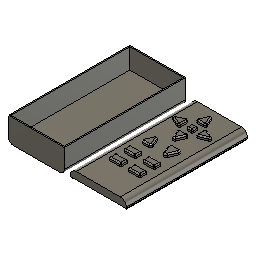
northreach_1_v1 (Autodesk Fusion 360 design; units mm, degrees)
Autodesk Fusion 360 part; units mm, degrees
sketch "Sketch1" plane through (0, 0, 0) normal (0, 1, 0) x (1, 0, 0)
  line L0 (-22.5, 50) -> (22.5, 50)
  line L1 (22.5, 50) -> (22.5, -50)
  line L2 (22.5, -50) -> (-22.5, -50)
  line L3 (-22.5, -50) -> (-22.5, 50)
  line L4 (-22.5, 50) -> (22.5, -50) construction
  line L5 (22.5, 50) -> (-22.5, -50) construction
  line L6 (-23.5, 51) -> (23.5, 51)
  line L7 (23.5, 51) -> (23.5, -51)
  line L8 (23.5, -51) -> (-23.5, -51)
  line L9 (-23.5, -51) -> (-23.5, 51)
  line L10 (-23.5, 51) -> (23.5, -51) construction
  line L11 (23.5, 51) -> (-23.5, -51) construction
  dimension "d1" = 45
  dimension "d2" = 100
  dimension "d3" = 47
  dimension "d4" = 102
  constraint horizontal L0
  constraint perpendicular L0 L1
  constraint parallel L0 L2
  constraint parallel L1 L3
  constraint coincident L4 origin
  constraint coincident L5 origin
  constraint horizontal L6
  constraint perpendicular L6 L7
  constraint parallel L6 L8
  constraint parallel L7 L9
  constraint coincident L10 origin
  constraint coincident L11 origin
  measures "d1" distance of L1.end L2.end
  measures "d2" distance of L0.end L1.end
  measures "d3" distance of L7.end L8.end
  measures "d4" distance of L6.end L7.end
extrude "Extrude1" add sketch "Sketch1" along normal blind 3 contours L0 L1 L2 L3 makes body 1
extrude "Extrude2" add sketch "Sketch1" along normal blind 20 bodies 1
fillet "Fillet1" radius 4 2 edges at (-23.5, 0, 0) (23.5, 0, 0) on bodies 1
sketch "Sketch4" plane through (0, 0, 0) normal (0, 1, 0) x (1, 0, 0)
  line L0 (46.5, 51) -> (93.5, 51)
  line L1 (93.5, 51) -> (93.5, -51)
  line L2 (93.5, -51) -> (46.5, -51)
  line L3 (46.5, -51) -> (46.5, 51)
  line L4 (46.5, 51) -> (93.5, -51) construction
  line L5 (93.5, 51) -> (46.5, -51) construction
  line L6 (48.5, 50) -> (91.5, 50)
  line L7 (91.5, 50) -> (91.5, -50)
  line L8 (91.5, -50) -> (48.5, -50)
  line L9 (48.5, -50) -> (48.5, 50)
  line L10 (48.5, 50) -> (91.5, -50) construction
  line L11 (91.5, 50) -> (48.5, -50) construction
  line L12 (48.5, 50) -> (47.5, 50)
  line L13 (47.5, 50) -> (47.5, -50)
  line L14 (47.5, -50) -> (48.5, -50)
  line L15 (48.5, -50) -> (48.5, 50)
  line L16 (91.5, -50) -> (92.5, -50)
  line L17 (92.5, -50) -> (92.5, 50)
  line L18 (92.5, 50) -> (91.5, 50)
  line L19 (91.5, 50) -> (91.5, -50)
  point P0 (70, 0)
  point P1 (70, 0)
  dimension "d22" = 47
  dimension "d23" = 102
  dimension "d24" = 43
  dimension "d25" = 100
  constraint horizontal L0
  constraint perpendicular L0 L1
  constraint parallel L0 L2
  constraint parallel L1 L3
  constraint coincident L4 P1
  constraint coincident L5 P1
  constraint horizontal L6
  constraint perpendicular L6 L7
  constraint parallel L6 L8
  constraint parallel L7 L9
  constraint coincident L10 P1
  constraint coincident L11 P1
  constraint coincident P1 P0
  constraint horizontal L12
  constraint vertical L13
  constraint horizontal L14
  constraint vertical L15
  constraint horizontal L16
  constraint vertical L17
  constraint horizontal L18
  constraint vertical L19
  measures "d22" distance of L1.end L2.end
  measures "d23" distance of L0.end L1.end
  measures "d24" distance of L7.end L8.end
  measures "d25" distance of L6.end L7.end
extrude "Extrude7" add sketch "Sketch4" along normal blind 2 separate body contours L6 L7 L8 L9 L15 L19 makes body 2
extrude "Extrude8" add sketch "Sketch4" along normal blind 6 bodies 2
extrude "Extrude9" add sketch "Sketch4" along normal blind 7.5 contours L9 L12 L13 L14 L15 | L7 L16 L17 L18 L19 bodies 2
fillet "Fillet2" radius 5 4 edges at (91.5, 2, 0) (48.5, 2, 0) (46.5, 0, 0) (93.5, 0, 0) on bodies 2
move_body "Move1" bodies 2 to x (-1, 0, 0) y (0, -1, 0) z (0, 0, 1) at (122, 7.5, 0)
sketch "Sketch5" plane through (0, 7.5, 0) normal (0, 1, 0) x (-1, 0, 0)
  line L0 (-33.5, -51) -> (-33.5, 51)
  line L1 (-33.5, 51) -> (-70.5, 51)
  line L2 (-70.5, 51) -> (-70.5, -51)
  line L3 (-70.5, -51) -> (-33.5, -51)
  arc A0 (-59.0385, -25.2061) -> (-60.6066, -24.1721) centre (-60.1635, -25.2061) ccw
  arc A1 (-39, 16.25) -> (-39.75, 17) centre (-39.75, 16.25) ccw
  line L4 (-49, 14) -> (-55, 14)
  arc A2 (-50.25, -30.5) -> (-49.5, -29.75) centre (-50.25, -29.75) ccw
  line L5 (-39.75, 11) -> (-48.25, 11)
  arc A3 (-55, 16.25) -> (-55.75, 17) centre (-55.75, 16.25) ccw
  line L6 (-46, 14) -> (-42, 14)
  line L7 (-53.75, -30.5) -> (-50.25, -30.5)
  arc A4 (-36.8743, -29.034) -> (-36.8743, -26.966) centre (-37.3174, -28) ccw
  line L8 (-54.5, -26.25) -> (-54.5, -29.75)
  line L9 (-49.5, -25.5) -> (-54.5, -30.5) construction
  arc A5 (-65, 11.75) -> (-64.25, 11) centre (-64.25, 11.75) ccw
  arc A6 (-49.2061, -20.9615) -> (-48.1721, -19.3934) centre (-49.2061, -19.8365) ccw
  line L10 (-65, 11) -> (-55, 17) construction
  line L11 (-39, 16.25) -> (-39, 11.75)
  line L12 (-48.25, 17) -> (-39.75, 17)
  line L13 (-65, 23) -> (-55, 29) construction
  line L14 (-62, 26) -> (-58, 26)
  line L15 (-41.4931, 3.0384) -> (-46.5069, 3.0384)
  line L16 (-39, 28.25) -> (-39, 23.75)
  arc A7 (-57.46, -6.6101) -> (-55.6908, -3.9272) centre (-57.46, -4.6854) ccw
  line L17 (-55.75, 23) -> (-64.25, 23)
  arc A8 (-39.75, 11) -> (-39, 11.75) centre (-39.75, 11.75) ccw
  line L18 (-49, 23) -> (-39, 29) construction
  line L19 (-39.75, 23) -> (-48.25, 23)
  arc A9 (-64.25, 29) -> (-65, 28.25) centre (-64.25, 28.25) ccw
  line L20 (-60, -6.6101) -> (-60, 3.4562)
  arc A10 (-64.3092, -3.9272) -> (-62.54, -6.6101) centre (-62.54, -4.6854) ccw
  arc A11 (-48.1721, -36.6066) -> (-49.2061, -35.0385) centre (-49.2061, -36.1635) ccw
  line L21 (-55, 11) -> (-65, 17) construction
  arc A12 (-49.5, -26.25) -> (-50.25, -25.5) centre (-50.25, -26.25) ccw
  line L22 (-49, 11) -> (-39, 17) construction
  arc A13 (-54.7939, -35.0385) -> (-55.8279, -36.6066) centre (-54.7939, -36.1635) ccw
  arc A14 (-49, 23.75) -> (-48.25, 23) centre (-48.25, 23.75) ccw
  line L23 (-47.8763, 0.9617) -> (-45.1295, -5.4475)
  arc A15 (-50.966, -12.8743) -> (-53.034, -12.8743) centre (-52, -13.3174) ccw
  line L24 (-58.4041, 2.4038) -> (-55.6908, -3.9272)
  arc A16 (-55.8279, -19.3934) -> (-54.7939, -20.9615) centre (-54.7939, -19.8365) ccw
  line L25 (-55, 28.25) -> (-55, 23.75)
  line L26 (-36.8743, -29.034) -> (-43.3934, -31.8279)
  arc A17 (-67.1257, -26.966) -> (-67.1257, -29.034) centre (-66.6826, -28) ccw
  line L27 (-49, 26) -> (-55, 26)
  line L28 (-57.46, -6.6101) -> (-62.54, -6.6101)
  line L29 (-50.966, -12.8743) -> (-48.1721, -19.3934)
  arc A18 (-47.8763, 0.9617) -> (-46.5069, 3.0384) centre (-46.5069, 1.5486) cw
  arc A19 (-58.4041, 2.4038) -> (-61.5959, 2.4038) centre (-60, 1.7199) ccw
  line L30 (-42.8705, -5.4475) -> (-40.1237, 0.9617)
  arc A20 (-36.8743, -29.034) -> (-36.8743, -26.966) centre (-37.3174, -28) ccw
  line L31 (-55, 23) -> (-65, 29) construction
  arc A21 (-55, 28.25) -> (-55.75, 29) centre (-55.75, 28.25) ccw
  line L32 (-54.5, -25.5) -> (-49.5, -30.5) construction
  line L33 (-36.8743, -29.034) -> (-43.3934, -31.8279)
  line L34 (-44.9615, -30.7939) -> (-44.9615, -25.2061)
  arc A22 (-44.9615, -30.7939) -> (-43.3934, -31.8279) centre (-43.8365, -30.7939) ccw
  line L35 (-65, 23.75) -> (-65, 28.25)
  line L36 (-46, 26) -> (-42, 26)
  line L37 (-64.25, 17) -> (-55.75, 17)
  line L38 (-59.0385, -25.2061) -> (-59.0385, -30.7939)
  line L39 (-39, 11) -> (-49, 17) construction
  arc A23 (-54.5, -29.75) -> (-53.75, -30.5) centre (-53.75, -29.75) ccw
  line L40 (-67.1257, -26.966) -> (-60.6066, -24.1721)
  line L41 (-43.3934, -24.1721) -> (-36.8743, -26.966)
  line L42 (-60.6066, -31.8279) -> (-67.1257, -29.034)
  line L43 (-50.25, -25.5) -> (-53.75, -25.5)
  arc A24 (-53.75, -25.5) -> (-54.5, -26.25) centre (-53.75, -26.25) ccw
  line L44 (-48.1721, -36.6066) -> (-50.966, -43.1257)
  line L45 (-49.2061, -20.9615) -> (-54.7939, -20.9615)
  line L46 (-44, 12) -> (-44, 16)
  arc A25 (-49, 11.75) -> (-48.25, 11) centre (-48.25, 11.75) ccw
  line L47 (-60, 24) -> (-60, 28)
  line L48 (-65, 11.75) -> (-65, 16.25)
  line L49 (-44, 24) -> (-44, 28)
  line L50 (-39, 23) -> (-49, 29) construction
  arc A26 (-43.3934, -24.1721) -> (-44.9615, -25.2061) centre (-43.8365, -25.2061) ccw
  line L51 (-62, 14) -> (-58, 14)
  line L52 (-49.5, -29.75) -> (-49.5, -26.25)
  line L53 (-60, 12) -> (-60, 16)
  arc A27 (-64.25, 17) -> (-65, 16.25) centre (-64.25, 16.25) ccw
  line L54 (-49, 11.75) -> (-49, 16.25)
  arc A28 (-65, 23.75) -> (-64.25, 23) centre (-64.25, 23.75) ccw
  arc A29 (-53.034, -43.1257) -> (-50.966, -43.1257) centre (-52, -42.6826) ccw
  arc A30 (-41.4931, 3.0384) -> (-40.1237, 0.9617) centre (-41.4931, 1.5486) cw
  arc A31 (-43.3934, -24.1721) -> (-44.9615, -25.2061) centre (-43.8365, -25.2061) ccw
  arc A32 (-48.25, 17) -> (-49, 16.25) centre (-48.25, 16.25) ccw
  arc A33 (-39, 28.25) -> (-39.75, 29) centre (-39.75, 28.25) ccw
  arc A34 (-44.9615, -30.7939) -> (-43.3934, -31.8279) centre (-43.8365, -30.7939) ccw
  line L55 (-44, -6.1923) -> (-44, 3.0384)
  line L56 (-49, 23.75) -> (-49, 28.25)
  line L57 (-43.3934, -24.1721) -> (-36.8743, -26.966)
  arc A35 (-55.75, 11) -> (-55, 11.75) centre (-55.75, 11.75) ccw
  arc A36 (-39.75, 23) -> (-39, 23.75) centre (-39.75, 23.75) ccw
  arc A37 (-60.6066, -31.8279) -> (-59.0385, -30.7939) centre (-60.1635, -30.7939) ccw
  line L58 (-48.25, 29) -> (-39.75, 29)
  line L59 (-54.7939, -35.0385) -> (-49.2061, -35.0385)
  line L60 (-55.75, 11) -> (-64.25, 11)
  line L61 (-44.9615, -30.7939) -> (-44.9615, -25.2061)
  line L62 (-55.8279, -19.3934) -> (-53.034, -12.8743)
  arc A38 (-48.25, 29) -> (-49, 28.25) centre (-48.25, 28.25) ccw
  line L63 (-53.034, -43.1257) -> (-55.8279, -36.6066)
  arc A39 (-42.8705, -5.4475) -> (-45.1295, -5.4475) centre (-44, -4.9635) cw
  line L64 (-64.3092, -3.9272) -> (-61.5959, 2.4038)
  line L65 (-64.25, 29) -> (-55.75, 29)
  arc A40 (-55.75, 23) -> (-55, 23.75) centre (-55.75, 23.75) ccw
  line L66 (-55, 16.25) -> (-55, 11.75)
  line L67 (-42, 16) -> (-46, 16) construction
  line L68 (-46, 16) -> (-46, 12) construction
  line L69 (-46, 12) -> (-42, 12) construction
  line L70 (-42, 12) -> (-42, 16) construction
  line L71 (-42, 28) -> (-46, 28) construction
  line L72 (-46, 28) -> (-46, 24) construction
  line L73 (-46, 24) -> (-42, 24) construction
  line L74 (-42, 24) -> (-42, 28) construction
  line L75 (-58, 16) -> (-62, 16) construction
  line L76 (-62, 16) -> (-62, 12) construction
  line L77 (-62, 12) -> (-58, 12) construction
  line L78 (-58, 12) -> (-58, 16) construction
  line L79 (-58, 28) -> (-62, 28) construction
  line L80 (-62, 28) -> (-62, 24) construction
  line L81 (-62, 24) -> (-58, 24) construction
  line L82 (-58, 24) -> (-58, 28) construction
  line L83 (-52, -35.0385) -> (-52, -43.8076)
  line L84 (-59.0385, -28) -> (-67.8076, -28)
  line L85 (-36.1924, -28) -> (-44.9615, -28)
  line L86 (-52, -20.9615) -> (-52, -12.1924)
  line L87 (-44, -1.577) -> (-60, -1.577)
  point P0 (-44, 26)
  point P1 (-60, 14)
  point P2 (-44, 3.0384)
  point P3 (-52.0007, 8.4459)
  point P4 (-44, 14)
  point P5 (-60, -6.6101)
  point P6 (-41.5, 10)
  point P7 (-44, 14)
  point P8 (-41.5, 22)
  point P9 (-44, 26)
  point P10 (-52, 14)
  point P11 (-60, -1.577)
  point P12 (-44, -1.577)
  point P13 (-52, 26)
  point P14 (-60, 14)
  point P15 (-52, -28)
  point P16 (-60, 26)
  point P17 (-60, 26)
  point P18 (-52, -39.423)
  point P19 (-63.423, -28)
  point P20 (-52, -16.577)
  point P21 (-40.577, -28)
  point P22 (-52, -1.577)
  dimension "d46" = 3
  dimension "d47" = 0
  dimension "d50" = 3
  dimension "d51" = 0
  dimension "d48" = 3
  dimension "d49" = 0
  dimension "d52" = 3
  dimension "d53" = 0
  dimension "d55" = 0.75
  dimension "d56" = 10
  dimension "d57" = 6
  dimension "d58" = 10
  dimension "d59" = 6
  dimension "d60" = 6
  dimension "d61" = 0.75
  dimension "d62" = 10
  dimension "d63" = 6
  dimension "d64" = 10
  dimension "d65" = 6
  dimension "d66" = 6
  dimension "d67" = 0.75
  dimension "d73" = 16
  text T0 "1" font "Arial" height 3 align centre middle in box 4 x 4 at (-42, 16) x (-1, 0) y (0, -1) spacing 1 kerned
  text T1 "3" font "Arial" height 3 align centre middle in box 4 x 4 at (-42, 28) x (-1, 0) y (0, -1) spacing 1 kerned
  text T2 "2" font "Arial" height 3 align centre middle in box 4 x 4 at (-58, 16) x (-1, 0) y (0, -1) spacing 1 kerned
  text T3 "4" font "Arial" height 3 align centre middle in box 4 x 4 at (-58, 28) x (-1, 0) y (0, -1) spacing 1 kerned
  constraint vertical L61
  constraint tangent L44 A29
  constraint tangent A29 L63
  constraint tangent A13 L59
  constraint tangent A13 L63
  constraint equal A13 A29
  constraint tangent A11 L44
  constraint tangent A11 L59
  constraint equal A11 A29
  constraint tangent A34 L61
  constraint tangent L33 A34
  constraint tangent A26 L61
  constraint tangent A26 L57
  constraint tangent A4 L57
  constraint tangent A4 L33
  constraint tangent L38 A37
  constraint tangent L42 A37
  constraint tangent A0 L38
  constraint tangent A0 L40
  constraint tangent A17 L40
  constraint tangent A17 L42
  constraint tangent A16 L45
  constraint tangent A16 L62
  constraint tangent A6 L45
  constraint tangent A6 L29
  constraint tangent A15 L62
  constraint tangent A15 L29
  constraint vertical L34
  constraint tangent L34 A22
  constraint tangent L26 A22
  constraint tangent L34 A31
  constraint tangent L41 A31
  constraint tangent A20 L41
  constraint tangent L26 A20
  constraint horizontal L43
  constraint perpendicular L8 L43
  constraint parallel L7 L43
  constraint parallel L8 L52
  constraint coincident P15 L9
  constraint coincident P15 L32
  constraint coincident L9.end L7
  constraint coincident L9.end L8
  constraint tangent L7 A23
  constraint tangent L8 A23
  constraint coincident L32.end L7
  constraint coincident L32.end L52
  constraint tangent A2 L7
  constraint tangent A2 L52
  constraint equal A2 A23
  constraint coincident L9.start L52
  constraint coincident L9.start L43
  constraint tangent A12 L52
  constraint tangent A12 L43
  constraint equal A12 A23
  constraint coincident L32.start L43
  constraint coincident L32.start L8
  constraint tangent L43 A24
  constraint tangent L8 A24
  constraint equal A23 A24
  constraint tangent L15 A18
  constraint tangent L23 A18
  constraint tangent L15 A30
  constraint tangent L30 A30
  constraint tangent L23 A39
  constraint tangent L30 A39
  constraint midpoint P2 L15
  constraint tangent A10 L28
  constraint tangent A10 L64
  constraint tangent A7 L28
  constraint tangent A7 L24
  constraint tangent A19 L64
  constraint tangent L24 A19
  constraint midpoint P5 L28
  constraint midpoint L55.start A39
  constraint coincident P2 L55.end
  constraint perpendicular L15 L55
  constraint coincident P5 L20.start
  constraint midpoint L20.end A19
  constraint perpendicular L20 L28
  constraint midpoint P11 L20
  constraint midpoint P12 L55
  constraint horizontal L60
  constraint perpendicular L48 L60
  constraint parallel L37 L60
  constraint parallel L48 L66
  constraint horizontal L5
  constraint perpendicular L5 L54
  constraint parallel L5 L12
  constraint parallel L11 L54
  constraint midpoint P10 L4
  constraint tangent L11 A8
  constraint tangent L5 A8
  constraint tangent A1 L11
  constraint tangent A1 L12
  constraint equal A1 A8
  constraint coincident L4.start L54
  constraint tangent L12 A32
  constraint tangent L54 A32
  constraint equal A8 A32
  constraint tangent L5 A25
  constraint tangent A25 L54
  constraint equal A8 A25
  constraint coincident L4.end L66
  constraint coincident L21.start L66
  constraint tangent A35 L60
  constraint tangent A35 L66
  constraint equal A8 A35
  constraint coincident L10.end L66
  constraint tangent A3 L66
  constraint tangent A3 L37
  constraint equal A3 A8
  constraint coincident L21.end L37
  constraint tangent L37 A27
  constraint tangent L48 A27
  constraint equal A8 A27
  constraint tangent A5 L60
  constraint tangent A5 L48
  constraint equal A5 A8
  constraint horizontal L17
  constraint perpendicular L17 L35
  constraint parallel L17 L65
  constraint parallel L25 L35
  constraint horizontal L19
  constraint perpendicular L19 L56
  constraint parallel L19 L58
  constraint parallel L16 L56
  constraint midpoint P13 L27
  constraint tangent L16 A36
  constraint tangent L19 A36
  constraint tangent L16 A33
  constraint tangent A33 L58
  constraint equal A33 A36
  constraint coincident L27.start L56
  constraint tangent L58 A38
  constraint tangent L56 A38
  constraint equal A36 A38
  constraint tangent L19 A14
  constraint tangent A14 L56
  constraint equal A14 A36
  constraint coincident L27.end L25
  constraint coincident L31.start L25
  constraint tangent L17 A40
  constraint tangent L25 A40
  constraint equal A36 A40
  constraint coincident L13.end L25
  constraint tangent L25 A21
  constraint tangent A21 L65
  constraint equal A21 A36
  constraint coincident L31.end L65
  constraint tangent A9 L65
  constraint tangent A9 L35
  constraint equal A9 A36
  constraint tangent L17 A28
  constraint tangent L35 A28
  constraint equal A28 A36
  constraint midpoint L46.start L69
  constraint midpoint L46.end L67
  constraint midpoint L6.start L68
  constraint midpoint L6.end L70
  constraint midpoint P7 L6
  constraint midpoint L53.start L77
  constraint midpoint L53.end L75
  constraint midpoint L51.start L76
  constraint midpoint L51.end L78
  constraint midpoint P14 L51
  constraint midpoint L49.start L73
  constraint midpoint L49.end L71
  constraint midpoint L36.start L72
  constraint midpoint L36.end L74
  constraint midpoint P9 L36
  constraint midpoint L47.start L81
  constraint midpoint L47.end L79
  constraint midpoint L14.start L80
  constraint midpoint L14.end L82
  constraint midpoint P17 L14
  constraint midpoint L59 L83.start
  constraint midpoint A29 L83.end
  constraint perpendicular L59 L83
  constraint midpoint L83 P18
  constraint midpoint L38 L84.start
  constraint midpoint A17 L84.end
  constraint perpendicular L38 L84
  constraint midpoint L84 P19
  constraint midpoint A20 L85.start
  constraint midpoint L34 L85.end
  constraint perpendicular L34 L85
  constraint midpoint L45 L86.start
  constraint midpoint A15 L86.end
  constraint perpendicular L45 L86
  constraint midpoint L86 P20
  constraint midpoint L85 P21
  constraint coincident P12 L87.start
  constraint coincident P11 L87.end
  constraint perpendicular L20 L87
  constraint midpoint L87 P22
  measures "d55" radius of A23
  measures "d56" distance of L21.end L10.end
  measures "d57" distance of L21.end L10.start
  measures "d58" distance of L22.end L39.end
  measures "d59" distance of L22.start L39.end
  measures "d60" distance of L54 L66
  measures "d61" radius of A8
  measures "d62" distance of L13.end L31.end
  measures "d63" distance of L13.start L31.end
  measures "d64" distance of L50.end L18.end
  measures "d65" distance of L50.end L18.start
  measures "d66" distance of L25 L56
  measures "d67" radius of A36
  measures "d73" distance of P12 P11
extrude "Extrude10" add sketch "Sketch5" sketch "Sketch5" along normal blind 2.5 contours A0 A17 L38 L40 L84 | A17 L38 L42 A37 L84 | A1 L5 L11 L12 A8 A25 L54 A32 | A2 L7 L8 A12 A23 L43 A24 L52 | A3 A5 L37 L48 A27 A35 L60 L66 | A4 L26 A20 L33 L34 A22 A34 L61 L85 | A4 A20 L34 L41 A26 A31 L57 L61 L85 | A6 A15 L29 L45 L86 | A15 A16 L45 L62 L86 | L15 L30 A30 L55 A39 | L15 L23 A18 L55 L87 | L23 L55 A39 L87 | L16 L19 A14 A33 L56 A36 L58 A38 | A7 L20 L24 L28 L87 | L20 A10 L28 A19 L64 | L20 L24 A19 L87 | L17 A9 L25 A21 L35 A28 L65 A40 | A11 L44 A29 L59 L83 | A13 A29 L59 L63 L83 of sketch 2 text T0 T1 T2 T3 bodies 2
fillet "Fillet3" radius 1 76 edges at (52, 10, -35.0385) (55.7331, 10, -35.5442) (54.431, 10, -39.8662) (52, 10, -43.8076) (49.569, 10, -39.8662) (48.2669, 10, -35.5442) (40.1338, 10, -25.569) (44.4558, 10, -24.2669) (44.9615, 10, -28) (44.4558, 10, -31.7331) (40.1338, 10, -30.431) (36.1924, 10, -28) (63.8662, 10, -25.569) (67.8076, 10, -28) (63.8662, 10, -30.431) (59.5442, 10, -31.7331) (59.0385, 10, -28) (59.5442, 10, -24.2669) (54.2803, 10, -30.2803) (52, 10, -30.5) (49.7197, 10, -30.2803) (49.5, 10, -28) (49.7197, 10, -25.7197) (52, 10, -25.5) (54.2803, 10, -25.7197) (54.5, 10, -28) (52, 10, -20.9615) (48.2669, 10, -20.4558) (49.569, 10, -16.1338) (52, 10, -12.1924) (54.431, 10, -16.1338) (55.7331, 10, -20.4558) (41.4971, 10, -2.2429) (40.2493, 10, 2.3687) (44, 10, 3.0384) (47.7507, 10, 2.3687) (46.5029, 10, -2.2429) (44, 10, -6.1923) (62.9525, 10, -0.7617) (64.1469, 10, -5.7449) (60, 10, -6.6101) (55.8531, 10, -5.7449) (57.0475, 10, -0.7617) (60, 10, 3.4562) (39, 10, 14) (39.2197, 10, 16.7803) (44, 10, 17) (48.7803, 10, 16.7803) (49, 10, 14) (48.7803, 10, 11.2197) (44, 10, 11) (39.2197, 10, 11.2197) (60, 10, 17) (64.7803, 10, 16.7803) (65, 10, 14) (64.7803, 10, 11.2197) (60, 10, 11) (55.2197, 10, 11.2197) (55, 10, 14) (55.2197, 10, 16.7803) (39, 10, 26) (39.2197, 10, 28.7803) (44, 10, 29) (48.7803, 10, 28.7803) (49, 10, 26) (48.7803, 10, 23.2197) (44, 10, 23) (39.2197, 10, 23.2197) (60, 10, 29) (64.7803, 10, 28.7803) (65, 10, 26) (64.7803, 10, 23.2197) (60, 10, 23) (55.2197, 10, 23.2197) (55, 10, 26) (55.2197, 10, 28.7803) on bodies 2
equation "d47 = '1'"
equation "d51 = '3'"
equation "d49 = '2'"
equation "d53 = '4'"
named bodies: "Main Body", "Top Cover"
